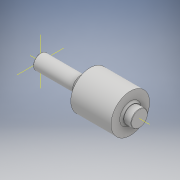
# Autodesk Inventor part: PogonskoVratilo
Saved by Autodesk Inventor 2018 (Build 220112000, 112)
## iProperties
Created: 2018-11-17
Part Number: PogonskoVratilo
Material: Generic
Document SubType Name: Modeling
Designer: Kristijan
Density: 1 g/cm^3
Appearance: Default
Author: Kristijan
Autodesk Inventor part; units mm, degrees
ref_plane "YZ Plane" through (0, 0, 0) normal (1, 0, 0) x (0, 1, 0)
ref_plane "XY Plane" through (0, 0, 0) normal (0, 0, 1) x (1, 0, 0)
sketch "Sketch1" plane through (0, 0, 0) normal (0, 0, 1) x (1, 0, 0)
  line L0 (0, 0) -> (0, 19)
  line L1 (1, 20) -> (110, 20)
  line L2 (110, 20) -> (110, 22.5)
  line L3 (110, 22.5) -> (130, 22.5)
  line L4 (130, 22.5) -> (130, 24)
  line L5 (130, 24) -> (130, 24)
  line L6 (135, 29) -> (135, 52.5)
  line L7 (135, 52.5) -> (245, 52.5)
  line L8 (245, 52.5) -> (245, 29)
  line L9 (250, 24) -> (250, 24)
  line L10 (250, 24) -> (250, 22.5)
  line L11 (250, 22.5) -> (269, 22.5)
  line L12 (270, 21.5) -> (270, 0)
  line L13 (270, 0) -> (0, 0)
  line L14 (0, 19) -> (1, 20)
  line L15 (269, 22.5) -> (270, 21.5)
  arc A0 (130, 24) -> (135, 29) centre (130, 29) ccw
  arc A1 (245, 29) -> (250, 24) centre (250, 29) ccw
  line L16 (-54, 0) -> (324, 0) projected
  point P0 (0, 20)
  point P1 (245, 24)
  point P2 (270, 22.5)
  dimension "d0" = 20
  dimension "d1" = 110
  dimension "d2" = 22.5
  dimension "d3" = 24
  dimension "d4" = 130
  dimension "d5" = 5
  dimension "d6" = 110
  dimension "d7" = 52.5
  dimension "d8" = 5
  dimension "d9" = 20
  dimension "d10" = 1
  dimension "d11" = 45
  dimension "d12" = 1
  dimension "d13" = 45
  dimension "d14" = 5
  constraints: 32 end point, 11 perpendicular, 10 point on line, 4 point on circle, 4 tangent, 2 centre point, 1 equal radius, 1 vertical
  measures "d0" distance between parallel lines of L13 L1
  measures "d1" distance between parallel lines of L2 L0
  measures "d2" distance between parallel lines of L13 L3
  measures "d3" distance between parallel lines of L13 L5
  measures "d4" distance between parallel lines of L4 L0
  measures "d5" distance between parallel lines of L6 L4
  measures "d6" distance of L6.end L7.end
  measures "d7" distance between parallel lines of L13 L7
  measures "d8" distance of point (245, 24) L9.end
  measures "d9" distance of L10.end point (270, 22.5)
  measures "d10" distance of L0.end point (0, 20)
  measures "d11" angle of L0 L14
  measures "d12" distance of L11.end point (270, 22.5)
  measures "d13" angle of L11 L15
  measures "d14" radius of A0
revolve "Revolution1" add sketch "Sketch1" angle 360 about axis through (-10, 0, 0) along (1, 0, 0)
ref_plane "Work Plane1" through (55.5, 20, 0) normal (0, 1, 0) x (-1, 0, 0)
sketch "Sketch2" plane through (55.5, 20, 0) normal (0, 1, 0) x (-1, 0, 0)
  line L0 (-44, 0) -> (44, 0) construction
  line L1 (-44, -6) -> (44, -6)
  line L2 (44, 6) -> (-44, 6)
  arc A0 (-44, 6) -> (-44, -6) centre (-44, 0) ccw
  arc A1 (44, -6) -> (44, 6) centre (44, 0) ccw
  point P0 (55.5, 0)
  point P1 (0, 0)
  dimension "d16" = 44
  dimension "d17" = 12
  constraints: 8 end point, 4 point on circle, 4 tangent, 2 centre point, 1 horizontal, 1 midpoint, 1 parallel
  measures "d16" distance of point (0, 0) L0.end
  measures "d17" diameter of A1
extrude "Extrusion1" cut sketch "Sketch2" against normal blind 5
equation "\"d8\" = d5"
equation "\"d12\" = d10"
equation "\"d13\" = d11"
body "Solid1"
